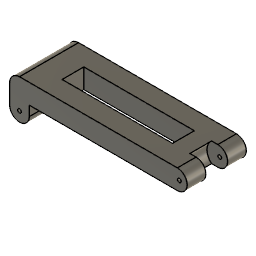
seminaire_FISA-A3_levier-poussoir (Autodesk Fusion 360 design; units mm, degrees)
part number: 2026-07-28-12-10-13-891
Autodesk Fusion 360 part; units mm, degrees
sketch "Esquisse1" plane through (0, 0, 0) normal (0, 0, 1) x (1, 0, 0)
  line L0 (-58.016, 25) -> (31.984, 25)
  line L1 (31.984, 25) -> (31.984, -5)
  line L2 (31.984, -5) -> (-58.016, -5)
  line L3 (-58.016, -5) -> (-58.016, 25)
  dimension "d1" = 90
  dimension "d2" = 30
  constraint horizontal L0
  constraint vertical L1
  constraint horizontal L2
  constraint vertical L3
  measures "d1" distance of L1.end L2.end
  measures "d2" distance of L0.end L1.end
extrude "Extrusion1" add sketch "Esquisse1" along normal blind 10
sketch "Esquisse11" plane through (0, 0, 0) normal (0, 1, 0) x (1, 0, 0)
  line L0 (-58.0163, -0.0111) -> (-48.0163, -0.0111)
  line L1 (-48.0163, -0.0111) -> (-48.0163, 9.9889)
  line L2 (-48.0163, 9.9889) -> (-58.0163, 9.9889)
  line L3 (-58.0163, 9.9889) -> (-58.0163, -0.0111)
  dimension "d56" = 10
  dimension "d57" = 10
  constraint horizontal L0
  constraint vertical L1
  constraint horizontal L2
  constraint vertical L3
  measures "d56" distance of L1.end L2.end
  measures "d57" distance of L0.start L2.end
extrude "Extrusion7" add sketch "Esquisse11" along normal blind 25 and the other way blind 5
sketch "Esquisse5" plane through (0, -5, 0) normal (0, -1, 0) x (1, 0, 0)
  line L0 (-48.0163, 0) -> (31.984, 0)
  line L1 (31.984, 0) -> (31.984, 10)
  line L2 (31.984, 10) -> (-58.016, 10)
  line L3 (-58.016, 10) -> (-58.016, 0.0111)
  circle A0 centre (28, 5) radius 6.5
  circle A1 centre (-53.0143, -5.2112) radius 7.25
  line L4 (-58.0163, 0.0111) -> (-58.0163, -9.9889)
  line L5 (-58.0163, -9.9889) -> (-48.0163, -9.9889)
  line L6 (-48.0163, -9.9889) -> (-48.0163, 0)
  line L7 (-58.016, 0.0111) -> (-58.0163, 0.0111)
  dimension "d11" = 13
  dimension "d46" = 14.5
  measures "d11" diameter of A0
  measures "d46" diameter of A1
sketch "Esquisse7" plane through (0, 0, 10) normal (0, 0, 1) x (-1, 0, 0)
  line L0 (-31.984, 5) -> (-31.984, -25)
  line L1 (-31.984, -25) -> (58.016, -25)
  line L2 (58.016, 5) -> (-31.984, 5)
  line L3 (41.016, -15.609) -> (-14.984, -15.609)
  line L4 (-14.984, -15.609) -> (-14.984, -4.609)
  line L5 (-14.984, -4.609) -> (41.016, -4.609)
  line L6 (41.016, -4.609) -> (41.016, -15.609)
  line L7 (58.016, -25) -> (58.016, 5)
  dimension "d47" = 11
  dimension "d48" = 56
  dimension "d49" = 17
  constraint horizontal L3
  constraint vertical L4
  constraint horizontal L5
  constraint vertical L6
  measures "d47" distance of L3.start L5.end
  measures "d48" distance of L3.start L3.end
  measures "d49" horizontal distance of L0.end L3.end
extrude "Extrusion9" cut sketch "Esquisse5" along normal blind -9.5 and the other way blind 20.5 contours L0 L3 A1 L4 L5 L6 | L0 L3 A1 L4 L5 L6 | L0 L1 L2 A0 picked at (28.4893, 5)
extrude "Extrusion4" cut sketch "Esquisse7" along normal blind 0 and the other way blind 10 contours L3 L4 L5 L6
sketch "Esquisse8" plane through (0, -5, 0) normal (0, -1, 0) x (1, 0, 0)
  line L0 (-48.0163, 0) -> (31.984, 0)
  line L1 (31.984, 0) -> (31.984, 10)
  line L2 (31.984, 10) -> (-58.016, 10)
  line L3 (-58.016, 10) -> (-58.016, 0.0111)
  circle A0 centre (-53, -5) radius 0.925
  line L4 (-58.016, 0.0111) -> (-58.0163, 0.0111)
  line L5 (-58.0163, 0.0111) -> (-58.0163, -9.9889)
  line L6 (-58.0163, -9.9889) -> (-48.0163, -9.9889)
  line L7 (-48.0163, -9.9889) -> (-48.0163, 0)
  dimension "d23" = 1.85
  measures "d23" diameter of A0
extrude "Extrusion5" cut sketch "Esquisse8" along normal blind 0 and the other way blind 30 contours A0
sketch "Esquisse9" plane through (0, -5, 0) normal (0, -1, 0) x (1, 0, 0)
  circle A0 centre (-53, -5) radius 0.925
  line L0 (-48.0163, 0) -> (31.984, 0)
  line L1 (31.984, 0) -> (31.984, 10)
  line L2 (31.984, 10) -> (-58.016, 10)
  line L3 (-58.016, 10) -> (-58.016, 0.0111)
  circle A1 centre (28, 5) radius 0.925
  line L4 (-58.016, 0.0111) -> (-58.0163, 0.0111)
  line L5 (-58.0163, 0.0111) -> (-58.0163, -9.9889)
  line L6 (-58.0163, -9.9889) -> (-48.0163, -9.9889)
  line L7 (-48.0163, -9.9889) -> (-48.0163, 0)
  dimension "d28" = 1.85
  measures "d28" diameter of A1
extrude "Extrusion6" cut sketch "Esquisse9" along normal blind 0 and the other way blind 30 contours A1
fillet "Congé8" radius 5 4 edges at (-58.0163, 20.25, -9.9889) (-58.0163, -0.25, -9.9889) (-48.0163, -0.25, -9.9889) (-48.0163, 20.25, -9.9889)
fillet "Congé9" radius 5 5 edges at (-58.016, 10, 10) (31.984, 20.25, 0) (31.984, -0.25, 0) (31.984, -0.25, 10) (31.984, 20.25, 10)
